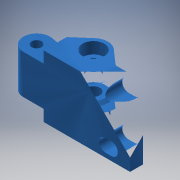
# Autodesk Inventor part: Infill3DIdler
Saved by Autodesk Inventor 2016 (Build 200138000, 138)
## iProperties
Created: 2015-04-27
Part Number: Infill3DIdler
Material: Generic
Document SubType Name: Modeling
Designer: Jack
Density: 1 g/cm^3
Appearance: Cyan
Author: Jack
Autodesk Inventor part; units mm, degrees
ref_plane "YZ Plane" through (0, 0, 0) normal (1, 0, 0) x (0, 1, 0)
sketch "Sketch1" plane through (0, 0, 0) normal (0, 0, 1) x (1, 0, 0)
  line L0 (0, 0) -> (30, 0)
  line L1 (30, 0) -> (30, 8)
  arc A0 (11.7951, 12.5606) -> (5.2049, 12.5606) centre (8.5, 8.8) ccw
  line L2 (30, 8) -> (17, 8)
  line L3 (0, 0) -> (0, 8)
  line L4 (0, 8) -> (5.2049, 12.5606)
  line L5 (11.7951, 12.5606) -> (17, 8)
  dimension "d0" = 8
  dimension "d1" = 30
  dimension "d3" = 8.8
  dimension "d4" = 10
  dimension "d5" = 8
  dimension "d56" = 8.5
  constraints: 12 end point, 2 horizontal, 2 point on circle, 2 tangent, 1 centre point, 1 equal length, 1 perpendicular, 1 vertical
  measures "d0" distance of L0.end L1.end
  measures "d1" distance of L0.start L0.end
  measures "d3" distance from line of L0 A0.centre
  measures "d4" diameter of A0
  measures "d5" distance of L0.start L3.end
  measures "d56" distance from line of L3 A0.centre
extrude "Extrusion1" add sketch "Sketch1" along normal blind 21.5
ref_plane "Work Plane1" through (0, 0, 10.75) normal (0, 0, 1) x (1, 0, 0)
sketch "Sketch2" plane through (0, 0, 10.75) normal (0, 0, 1) x (1, 0, 0)
  arc A0 (11.7951, 12.5606) -> (5.2049, 12.5606) centre (8.5, 8.8) ccw projected
  arc A1 (-6.1752, 9.1255) -> (-7, 0) centre (-7, 4.6) ccw
  line L0 (-6.1752, 9.1255) -> (0, 8)
  line L1 (-7, 0) -> (0, 0)
  line L2 (0, 8) -> (0, 0)
  dimension "d10" = 15.5
  dimension "d11" = 9.2
  constraints: 6 end point, 2 point on circle, 2 tangent, 1 centre point, 1 horizontal, 1 vertical
  measures "d10" horizontal distance of A1.centre A0.centre
  measures "d11" diameter of A1
extrude "Extrusion2" add sketch "Sketch2" along normal mid plane 13.6
sketch "Sketch3" plane through (0, 0, 17.55) normal (0, 0, 1) x (1, 0, 0)
  arc A0 (-6.1752, 9.1255) -> (-7, 0) centre (-7, 4.6) ccw projected
hole "Hole1" at (-7, 4.6, 17.55) direction (0, 0, -1) diameter 3.5 end through all
sketch "Sketch4" plane through (0, 0, 21.5) normal (0, 0, 1) x (1, 0, 0)
  arc A0 (11.7951, 12.5606) -> (5.2049, 12.5606) centre (8.5, 8.8) ccw projected
hole "Hole2" at (8.5, 8.8, 21.5) direction (0, 0, -1) diameter 4.5 end through all
ref_plane "Work Plane2" through (0, 0, 11.5) normal (0, 0, 1) x (1, 0, 0)
sketch "Sketch5" plane through (0, 0, 11.5) normal (0, 0, 1) x (1, 0, 0)
  circle A0 centre (8.5, 8.8) radius 2.25 projected
  circle A1 centre (8.5, 8.8) radius 8
  point P0 (0, 0)
  dimension "d29" = 16
  constraints: 1 centre point, 1 coincident
  measures "d29" diameter of A1
extrude "Extrusion3" cut sketch "Sketch5" along normal mid plane 7
sketch "Sketch6" plane through (0, 0, 21.5) normal (0, 0, 1) x (1, 0, 0)
  circle A0 centre (8.5, 8.8) radius 2.25 projected
hole "Hole3" at (8.5, 8.8, 21.5) direction (0, 0, -1) diameter 7.5 depth 4
sketch "Sketch8" plane through (0, 0, 8) normal (0, 0, 1) x (1, 0, 0)
  circle A0 centre (8.5, 8.8) radius 2.25 projected
  circle A1 centre (8.5, 8.8) radius 5
  point P0 (0, 0)
  dimension "d42" = 10
  constraints: 1 centre point, 1 coincident
  measures "d42" diameter of A1
extrude "Extrusion5" add sketch "Sketch8" along normal blind 1
sketch "Sketch9" plane through (0, 0, 15) normal (0, 0, -1) x (-1, 0, 0)
  arc A0 (-5.2049, 12.5606) -> (-11.7951, 12.5606) centre (-8.5, 8.8) ccw projected
  circle A1 centre (-8.5, 8.8) radius 2.25 projected
  circle A2 centre (-8.5, 8.8) radius 5
  point P0 (0, 0)
  constraints: 1 centre point, 1 coincident, 1 concentric
extrude "Extrusion6" add sketch "Sketch9" along normal blind 1
chamfer "Chamfer1" distance 1 angle 45 2 edges at (3.5, 8.8, 9) (13.5, 8.8, 14)
sketch "Sketch10" plane through (0, 0, 0) normal (0, -1, 0) x (1, 0, 0)
  line L0 (30, 0) -> (30, 21.5) projected
  line L1 (0, 21.5) -> (30, 21.5) projected
  line L2 (25.5, 17.75) -> (23.5, 17.75) construction
  line L3 (25.5, 20) -> (23.5, 20)
  line L4 (23.5, 15.5) -> (25.5, 15.5)
  arc A0 (25.5, 15.5) -> (25.5, 20) centre (25.5, 17.75) ccw
  arc A1 (23.5, 20) -> (23.5, 15.5) centre (23.5, 17.75) ccw
  line L5 (25.5, 3.75) -> (23.5, 3.75) construction
  line L6 (25.5, 6) -> (23.5, 6)
  line L7 (23.5, 1.5) -> (25.5, 1.5)
  arc A2 (25.5, 1.5) -> (25.5, 6) centre (25.5, 3.75) ccw
  arc A3 (23.5, 6) -> (23.5, 1.5) centre (23.5, 3.75) ccw
  point P0 (24.5, 17.75)
  point P1 (24.5, 3.75)
  dimension "d79" = 5.5
  dimension "d80" = 3.75
  dimension "d81" = 14
  dimension "d89" = 4.5
  dimension "d90" = 2
  constraints: 16 end point, 8 point on circle, 8 tangent, 4 centre point, 4 parallel, 2 midpoint, 1 equal radius, 1 horizontal, 1 vertical alignment
  measures "d79" distance from line of L0 point (24.5, 17.75)
  measures "d80" distance from line of L1 point (24.5, 17.75)
  measures "d81" distance of point (24.5, 3.75) point (24.5, 17.75)
  measures "d89" diameter of A1
  measures "d90" distance of L2.start L2.end
sketch "Sketch13" plane through (0, 0, 0) normal (0, 0, -1) x (-1, 0, 0)
  line L0 (-5.2049, 12.5606) -> (0, 8) projected
  arc A0 (-5.2049, 12.5606) -> (-11.7951, 12.5606) centre (-8.5, 8.8) ccw projected
  line L1 (-17, 8) -> (-11.7951, 12.5606) projected
  arc A1 (-14.4334, 10.2489) -> (-2.5666, 10.2489) centre (-8.5, 20.1) ccw
  dimension "d66" = 11.5
  dimension "d67" = 11.3
  constraints: 2 point on circle, 2 point on line, 1 centre point, 1 vertical alignment
  measures "d66" radius of A1
  measures "d67" distance of A0.centre A1.centre
extrude "Extrusion10" cut sketch "Sketch13" against normal blind 2.5
sketch "Sketch14" plane through (0, 0, 0) normal (0, 0, -1) x (-1, 0, 0)
  arc A0 (-10.7499, 8.8222) -> (-6.2501, 8.8222) centre (-8.5, 8.8) ccw projected
  line L0 (-8.5, 13.0724) -> (-4.8, 10.9362)
  line L1 (-4.8, 10.9362) -> (-4.8, 6.6638)
  line L2 (-4.8, 6.6638) -> (-8.5, 4.5276)
  line L3 (-8.5, 4.5276) -> (-12.2, 6.6638)
  line L4 (-12.2, 6.6638) -> (-12.2, 10.9362)
  line L5 (-12.2, 10.9362) -> (-8.5, 13.0724)
  dimension "d70" = 7.4
  constraints: 12 end point, 1 coincident, 1 vertical, 13 other
  measures "d70" distance between parallel lines of L1 L4
extrude "Extrusion11" cut sketch "Sketch14" against normal blind 6
chamfer "Chamfer3" distance 3.5 angle 45 1 edges at (30, 8, 10.75)
extrude "Extrusion12" cut sketch "Sketch10" against normal up to next
sketch "Sketch12" plane through (0, 0, 21.5) normal (0, 0, 1) x (1, 0, 0)
  line L0 (0, 0) -> (30, 0) projected
  line L1 (26, 0) -> (23.75, 0) projected
  line L2 (26, 0) -> (30, 0) projected
  arc A0 (27.6, 0) -> (24.4, 0) centre (26, -1.2) ccw
  dimension "d62" = 2
  dimension "d63" = 1.2
  constraints: 2 point on circle, 2 point on line, 1 centre point, 1 vertical alignment
  measures "d62" radius of A0
  measures "d63" distance from line of L0 A0.centre
body "Solid1"
